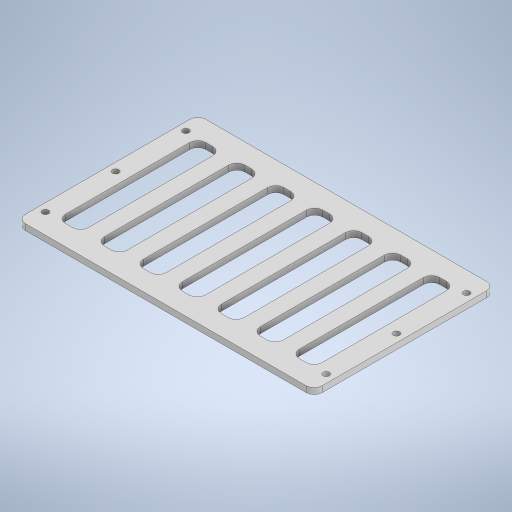
# Autodesk Inventor part: chest_cover_top
Saved by Autodesk Inventor 2024.1 (Build 281209000, 209)
## iProperties
Created: 2024-02-14
Part Number: chest_cover_top
Material: 一般
Document SubType Name: Modeling
Designer: hibik
Density: 1 g/cm^3
Appearance: 既定
Author: hibik
Autodesk Inventor part; units mm, degrees
ref_plane "YZ Plane" through (0, 0, 0) normal (1, 0, 0) x (0, 1, 0)
ref_plane "XZ Plane" through (0, 0, 0) normal (0, 1, 0) x (-1, 0, 0)
ref_plane "XY Plane" through (0, 0, 0) normal (0, 0, 1) x (1, 0, 0)
sketch "スケッチ1" plane through (0, 0, 0) normal (0, 1, 0) x (-1, 0, 0)
  line L0 (30, 0) -> (-30, 0)
  line L1 (-30, 0) -> (-30, -45)
  line L2 (-30, -45) -> (30, -45)
  line L3 (30, -45) -> (30, 0)
  line L4 (37, 0) -> (30, 0)
  line L5 (30, 0) -> (30, -45)
  line L6 (30, -45) -> (37, -45)
  line L7 (37, -45) -> (37, 0)
  line L8 (-30, 0) -> (-37, 0)
  line L9 (-37, 0) -> (-37, -45)
  line L10 (-37, -45) -> (-30, -45)
  line L11 (-30, -45) -> (-30, 0)
  line L12 (37, 0) -> (35, 0)
  line L13 (35, 0) -> (35, -45) construction
  line L14 (35, -45) -> (37, -45)
  line L15 (37, -45) -> (37, 0)
  line L16 (-37, 0) -> (-35, 0)
  line L17 (-35, 0) -> (-35, -45) construction
  line L18 (-35, -45) -> (-37, -45)
  line L19 (-37, -45) -> (-37, 0)
  circle A0 centre (35, -5) radius 0.8
  circle A1 centre (35, -40) radius 0.8
  circle A2 centre (-35, -5) radius 0.8
  circle A3 centre (-35, -40) radius 0.8
  circle A4 centre (-35, -22.5) radius 0.8
  circle A5 centre (35, -22.5) radius 0.8
  point P0 (0, 0)
  point P1 (0, 0)
  point P2 (30, 0)
  dimension "d0" = 60
  dimension "d1" = 45
  dimension "d4" = 7
  dimension "d5" = 2
  dimension "d6" = 2
  dimension "d7" = 1.6
  dimension "d8" = 1.6
  dimension "d9" = 1.6
  dimension "d10" = 1.6
  dimension "d11" = 5
  dimension "d12" = 5
  dimension "d13" = 1.6
  dimension "d14" = 1.6
  constraints: 40 end point, 10 parallel, 6 centre point, 6 point on line, 5 horizontal, 5 perpendicular, 3 collinear, 3 midpoint, 2 horizontal alignment, 1 coincident
  measures "d0" distance of L0.start L0.end
  measures "d1" distance of L2.end L0.start
  measures "d4" distance of L4.start L4.end
  measures "d5" distance between parallel lines of L15 L13
  measures "d6" distance between parallel lines of L19 L17
  measures "d7" diameter of A0
  measures "d8" diameter of A1
  measures "d9" diameter of A2
  measures "d10" diameter of A3
  measures "d11" distance from line of L8 A2.centre
  measures "d12" distance from line of L10 A3.centre
  measures "d13" diameter of A4
  measures "d14" diameter of A5
extrude "押し出し1" add sketch "スケッチ1" along normal blind 1.5
sketch "スケッチ2" plane through (0, 1.5, 0) normal (0, 1, 0) x (1, 0, 0)
  circle A0 centre (-35, 40) radius 0.8 projected
  circle A1 centre (35, 5) radius 0.8 projected
  line L0 (-35, 40) -> (35, 40)
  line L1 (35, 40) -> (35, 5)
  line L2 (35, 5) -> (-35, 5)
  line L3 (-35, 5) -> (-35, 40)
  line L4 (-32, 40) -> (32, 40)
  line L5 (32, 40) -> (32, 5)
  line L6 (32, 5) -> (-32, 5)
  line L7 (-32, 5) -> (-32, 40)
  line L8 (-26.2857, 40) -> (-22.2857, 40)
  line L9 (-22.2857, 40) -> (-22.2857, 5)
  line L10 (-22.2857, 5) -> (-26.2857, 5)
  line L11 (-26.2857, 5) -> (-26.2857, 40)
  line L12 (-16.5714, 40) -> (-12.5714, 40)
  line L13 (-12.5714, 40) -> (-12.5714, 5)
  line L14 (-12.5714, 5) -> (-16.5714, 5)
  line L15 (-16.5714, 5) -> (-16.5714, 40)
  line L16 (-6.8571, 40) -> (-2.8571, 40)
  line L17 (-2.8571, 40) -> (-2.8571, 5)
  line L18 (-2.8571, 5) -> (-6.8571, 5)
  line L19 (-6.8571, 5) -> (-6.8571, 40)
  line L20 (2.8571, 40) -> (6.8571, 40)
  line L21 (6.8571, 40) -> (6.8571, 5)
  line L22 (6.8571, 5) -> (2.8571, 5)
  line L23 (2.8571, 5) -> (2.8571, 40)
  line L24 (12.5714, 40) -> (16.5714, 40)
  line L25 (16.5714, 40) -> (16.5714, 5)
  line L26 (16.5714, 5) -> (12.5714, 5)
  line L27 (12.5714, 5) -> (12.5714, 40)
  line L28 (22.2857, 40) -> (26.2857, 40)
  line L29 (26.2857, 40) -> (26.2857, 5)
  line L30 (26.2857, 5) -> (22.2857, 5)
  line L31 (22.2857, 5) -> (22.2857, 40)
  point P0 (0, 0)
  point P1 (32, 40)
  point P2 (6.8571, 5)
  dimension "d16" = 3
  dimension "d17" = 3
  dimension "d18" = 4
  dimension "d19" = 5.7143
  dimension "d20" = 5.7143
  dimension "d21" = 5.7143
  dimension "d22" = 5.7143
  dimension "d23" = 5.7143
  dimension "d24" = 5.7143
  dimension "d25" = 5.7143
  constraints: 64 end point, 16 parallel, 10 collinear, 9 point on line, 8 horizontal, 8 perpendicular
  measures "d16" distance between parallel lines of L3 L7
  measures "d17" distance between parallel lines of L1 L5
  measures "d18" distance of L9.end L10.end
  measures "d19" distance between parallel lines of L11 L7
  measures "d20" distance between parallel lines of L15 L9
  measures "d21" distance between parallel lines of L19 L13
  measures "d22" distance between parallel lines of L23 L17
  measures "d23" distance between parallel lines of L27 L21
  measures "d24" distance between parallel lines of L31 L25
  measures "d25" distance between parallel lines of L5 L29
extrude "押し出し2" cut sketch "スケッチ2" against normal through all contours L0 L11 L2 L7 | L0 L15 L2 L9 | L0 L19 L2 L13 | L0 L23 L2 L17 | L0 L27 L2 L21 | L0 L31 L2 L25 | L0 L5 L2 L29
fillet "フィレット1" radius 2 32 edges at (-37, 0.75, 0) (-37, 0.75, -45) (37, 0.75, 0) (37, 0.75, -45) (-32, 0.75, -40) (-22.2857, 0.75, -40) (-12.5714, 0.75, -40) (-2.8571, 0.75, -40) (6.8571, 0.75, -40) (16.5714, 0.75, -40) (26.2857, 0.75, -40) (32, 0.75, -40) (22.2857, 0.75, -40) (12.5714, 0.75, -40) (2.8571, 0.75, -40) (-6.8571, 0.75, -40) (-16.5714, 0.75, -40) (-26.2857, 0.75, -40) (-26.2857, 0.75, -5) (-16.5714, 0.75, -5) (-6.8571, 0.75, -5) (2.8571, 0.75, -5) (12.5714, 0.75, -5) (22.2857, 0.75, -5) (32, 0.75, -5) (-32, 0.75, -5) (-22.2857, 0.75, -5) (-12.5714, 0.75, -5) (-2.8571, 0.75, -5) (6.8571, 0.75, -5) (16.5714, 0.75, -5) (26.2857, 0.75, -5)
equation "\"d19\" = d25"
equation "\"d20\" = d25"
equation "\"d21\" = d25"
equation "\"d22\" = d25"
equation "\"d23\" = d25"
equation "\"d24\" = d25"
